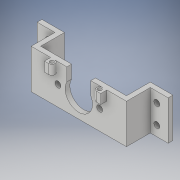
# Autodesk Inventor part: yaxis_clamp2
Saved by Autodesk Inventor 2019 (Build 230136000, 136)
## iProperties
Created: 2020-02-02
Material: Generic
Document SubType Name: Modeling
Designer: Nishant
Density: 1 g/cm^3
Appearance: Default
Author: Nishant
Autodesk Inventor part; units mm, degrees
ref_plane "YZ Plane" through (0, 0, 0) normal (1, 0, 0) x (0, 1, 0)
ref_plane "XZ Plane" through (0, 0, 0) normal (0, 1, 0) x (-1, 0, 0)
ref_plane "XY Plane" through (0, 0, 0) normal (0, 0, 1) x (1, 0, 0)
sketch "Sketch1" plane through (0, 0, 0) normal (0, 0, 1) x (1, 0, 0)
  line L0 (0, 0) -> (0, 33)
  line L1 (0, 33) -> (19, 33)
  line L2 (19, 33) -> (19, 0)
  line L3 (19, 0) -> (0, 0)
  dimension "d0" = 33
  dimension "d1" = 19
  constraints: 8 end point, 2 perpendicular, 2 vertical
  measures "d0" distance of L0.start L0.end
  measures "d1" distance of L0.end L1.end
extrude "Extrusion1" add sketch "Sketch1" along normal blind 4
sketch "Sketch2" plane through (0, 33, 0) normal (0, 1, 0) x (1, 0, 0)
  line L0 (19, 0) -> (0, 0) projected
  line L1 (19, 0) -> (19, -24)
  line L2 (19, -24) -> (15, -24)
  line L3 (15, -24) -> (15, 0)
  line L4 (15, 0) -> (19, 0)
  dimension "d4" = 24
  dimension "d5" = 4
  dimension "d6" = 24
  constraints: 8 end point, 1 perpendicular, 1 point on line, 1 vertical
  measures "d4" distance of L0.start L1.end
  measures "d5" distance of L1.end L2.end
  measures "d6" distance of L2.end L3.end
extrude "Extrusion2" add sketch "Sketch2" against normal blind 33
sketch "Sketch3" plane through (0, 33, 0) normal (0, 1, 0) x (1, 0, 0)
  line L0 (15, -4) -> (15, -24) projected
  line L1 (15, -24) -> (95, -24)
  line L2 (95, -24) -> (95, -20)
  line L3 (95, -20) -> (15, -20)
  line L4 (15, -20) -> (15, -24)
  point P0 (0, 0)
  dimension "d9" = 80
  dimension "d10" = 4
  dimension "d11" = 80
  constraints: 8 end point, 1 horizontal, 1 perpendicular, 1 point on line, 1 vertical
  measures "d9" distance of L0.end L1.end
  measures "d10" distance of L1.end L2.end
  measures "d11" distance of L2.end L3.end
extrude "Extrusion3" add sketch "Sketch3" against normal blind 33
sketch "Sketch4" plane through (0, 33, 0) normal (0, 1, 0) x (1, 0, 0)
  line L0 (15, -24) -> (95, -24) projected
  line L1 (95, -24) -> (95, 0)
  line L2 (95, 0) -> (91, 0)
  line L3 (91, 0) -> (91, -24)
  line L4 (91, -24) -> (95, -24)
  point P0 (0, 0)
  dimension "d14" = 24
  dimension "d15" = 4
  dimension "d16" = 24
  constraints: 8 end point, 1 collinear, 1 perpendicular, 1 point on line, 1 vertical
  measures "d14" distance of L0.end L1.end
  measures "d15" distance of L1.end L2.end
  measures "d16" distance of L2.end L3.end
extrude "Extrusion4" add sketch "Sketch4" against normal blind 33
sketch "Sketch5" plane through (0, 33, 0) normal (0, 1, 0) x (1, 0, 0)
  line L0 (91, 0) -> (91, -20) projected
  line L1 (91, 0) -> (110, 0)
  line L2 (110, 0) -> (110, -4)
  line L3 (110, -4) -> (91, -4)
  line L4 (91, -4) -> (91, 0)
  point P0 (0, 0)
  dimension "d19" = 19
  dimension "d20" = 4
  dimension "d21" = 19
  dimension "d22" = 4
  constraints: 8 end point, 1 collinear, 1 horizontal, 1 perpendicular, 1 point on line
  measures "d19" distance of L0.start L1.end
  measures "d20" distance of L1.end L2.end
  measures "d21" distance of L2.end L3.end
  measures "d22" distance of L3.end L0.start
extrude "Extrusion5" add sketch "Sketch5" against normal blind 33
sketch "Sketch6" plane through (15, 0, 24) normal (0, 0, 1) x (1, 0, 0)
  line L0 (80, 33) -> (80, 0) projected
  line L1 (30, 33) -> (30, 22.18)
  line L2 (50, 33) -> (50, 22.18)
  arc A0 (30.0006, 22.18) -> (49.9994, 22.18) centre (40, 16.5) ccw
  line L3 (30, 22.18) -> (30.0006, 22.18)
  line L4 (49.9994, 22.18) -> (50, 22.18)
  line L5 (30, 33) -> (50, 33)
  line L6 (0, 33) -> (80, 33) projected
  point P0 (-15, 0)
  dimension "d27" = 10.82
  dimension "d28" = 10.82
  dimension "d30" = 23
  constraints: 10 end point, 2 horizontal, 2 point on circle, 2 vertical, 1 centre point, 1 collinear
  measures "d27" distance of L1.start L1.end
  measures "d28" distance of L2.start L2.end
  measures "d30" diameter of A0
extrude "Extrusion6" cut sketch "Sketch6" against normal blind 4
sketch "Sketch7" plane through (0, 0, 0) normal (0, 0, -1) x (-1, 0, 0)
  line L0 (0, 33) -> (-19, 33) projected
  line L1 (-19, 0) -> (0, 0) projected
  circle A0 centre (-9.5, 24.5) radius 2.5
  circle A1 centre (-9.5, 8.5) radius 2.5
  dimension "d35" = 5
  dimension "d36" = 5
  constraints: 2 centre point
  measures "d35" diameter of A0
  measures "d36" diameter of A1
extrude "Extrusion7" cut sketch "Sketch7" against normal blind 4
sketch "Sketch8" plane through (91, 0, 0) normal (0, 0, -1) x (-1, 0, 0)
  circle A0 centre (-9.5, 24.5) radius 2.5
  circle A1 centre (-9.5, 8.5) radius 2.5
  point P0 (91, 0)
  point P1 (-19, 33)
  point P2 (0, 33)
  point P3 (-19, 0)
  point P4 (0, 0)
  dimension "d39" = 19
  dimension "d43" = 5
  dimension "d44" = 5
  constraints: 2 centre point
  measures "d39" distance of point (-19, 33) point (0, 33)
  measures "d43" diameter of A0
  measures "d44" diameter of A1
extrude "Extrusion8" cut sketch "Sketch8" against normal blind 4
sketch "Sketch9" plane through (15, 0, 24) normal (0, 0, 1) x (1, 0, 0)
  line L0 (0, 33) -> (30, 33) projected
  line L1 (0, 0) -> (0, 33) projected
  circle A0 centre (22.5, 16.5) radius 2.5
  line L2 (50, 33) -> (80, 33) projected
  line L3 (80, 0) -> (80, 33) projected
  circle A1 centre (57.5, 16.5) radius 2.5
  point P0 (-15, 0)
  dimension "d49" = 5
  dimension "d52" = 5
  constraints: 2 centre point
  measures "d49" diameter of A0
  measures "d52" diameter of A1
extrude "Extrusion9" cut sketch "Sketch9" against normal blind 4
sketch "Sketch10" plane through (0, 33, 0) normal (0, 1, 0) x (1, 0, 0)
  line L0 (31.4, -24) -> (31.4, -29.2)
  line L1 (31.4, -29.2) -> (35, -29.2)
  line L2 (37.6, -26.6) -> (37.6, -26.6)
  line L3 (40, -24) -> (35, -24) projected
  line L4 (35, -24) -> (31.4, -24)
  arc A0 (37.6, -26.6) -> (35, -24) centre (35, -26.6) ccw
  arc A1 (35, -29.2) -> (37.6, -26.6) centre (35, -26.6) ccw
  circle A2 centre (35, -26.6) radius 1.6
  point P0 (0, 0)
  point P1 (15, -24)
  point P2 (37.6, -29.2)
  point P3 (37.6, -24)
  dimension "d56" = 5.2
  dimension "d57" = 6.2
  dimension "d58" = 5.2
  dimension "d59" = 6.2
  dimension "d60" = 2.6
  dimension "d61" = 3.2
  constraints: 8 end point, 5 point on line, 4 point on circle, 4 tangent, 3 centre point, 1 coincident, 1 concentric, 1 horizontal
  measures "d56" distance of L0.start L0.end
  measures "d57" distance of L0.end point (37.6, -29.2)
  measures "d58" distance of point (37.6, -29.2) point (37.6, -24)
  measures "d59" distance of point (37.6, -24) L0.start
  measures "d60" radius of A0
  measures "d61" diameter of A2
extrude "Extrusion10" add sketch "Sketch10" against normal blind 8
sketch "Sketch11" plane through (91, 33, 20) normal (0, 1, 0) x (1, 0, 0)
  line L0 (-12.4, -4) -> (-12.4, -9.2)
  line L1 (-12.4, -9.2) -> (-16, -9.2)
  line L2 (-18.6, -6.6) -> (-18.6, -6.6)
  line L3 (-16, -4) -> (-21, -4) projected
  line L4 (-16, -4) -> (-12.4, -4)
  arc A0 (-16, -4) -> (-18.6, -6.6) centre (-16, -6.6) ccw
  arc A1 (-18.6, -6.6) -> (-16, -9.2) centre (-16, -6.6) ccw
  circle A2 centre (-16, -6.6) radius 1.6
  point P0 (-91, 20)
  point P1 (4, -4)
  point P2 (-18.6, -9.2)
  point P3 (-18.6, -4)
  dimension "d64" = 16.4
  dimension "d65" = 5.2
  dimension "d66" = 6.2
  dimension "d67" = 5.2
  dimension "d68" = 6.2
  dimension "d69" = 2.6
  dimension "d70" = 3.2
  constraints: 8 end point, 5 point on line, 4 point on circle, 4 tangent, 3 centre point, 1 coincident, 1 concentric, 1 perpendicular, 1 vertical
  measures "d64" distance of point (4, -4) L0.start
  measures "d65" distance of L0.start L0.end
  measures "d66" distance of L0.end point (-18.6, -9.2)
  measures "d67" distance of point (-18.6, -9.2) point (-18.6, -4)
  measures "d68" distance of point (-18.6, -4) L0.start
  measures "d69" radius of A0
  measures "d70" diameter of A2
extrude "Extrusion11" add sketch "Sketch11" against normal blind 8
body "Solid1"
